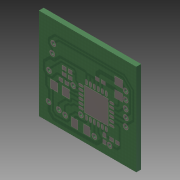
# Autodesk Inventor part: LED_module_PCB
Saved by Autodesk Inventor 2013 (Build 170138000, 138)
## iProperties
Created: 2015-07-03
Part Number: LED_module_PCB
Material: Ogólny
Document SubType Name: Modeling
Designer: terg
Density: 1 g/cm^3
Author: terg
Autodesk Inventor part; units mm, degrees
ref_plane "YZ Plane" through (0, 0, 0) normal (1, 0, 0) x (0, 1, 0)
ref_plane "XZ Plane" through (0, 0, 0) normal (0, 1, 0) x (-1, 0, 0)
ref_plane "XY Plane" through (0, 0, 0) normal (0, 0, 1) x (1, 0, 0)
sketch "Szkic1" plane through (0, 0, 0) normal (0, 1, 0) x (-1, 0, 0)
  line L0 (0, 0) -> (16, 0)
  line L1 (16, 0) -> (16, 15)
  line L2 (16, 15) -> (0, 15)
  line L3 (0, 15) -> (0, 0)
  dimension "d0" = 16
  dimension "d1" = 15
  constraints: 8 end point, 2 parallel, 1 horizontal, 1 perpendicular
  measures "d0" distance of L2.end L1.end
  measures "d1" distance of L1.end L0.end
extrude "Wyciągnięcie proste1" add sketch "Szkic1" along normal blind 0.8
sketch "Szkic2" plane through (0, 0.8, 0) normal (0, 1, 0) x (1, 0, 0)
  line L0 (0, 0) -> (-16, 0) projected
  line L1 (-16, 0) -> (-16, -15) projected
  line L2 (-16, -15) -> (0, -15) projected
  line L3 (0, -15) -> (0, 0) projected
  line L4 (-16.025, 0) -> (0.025, 0) construction
  line L5 (0.025, 0) -> (0.025, -15) construction
  line L6 (0.025, -15) -> (-16.025, -15) construction
  line L7 (-16.025, -15) -> (-16.025, 0) construction
  dimension "d11" = -0.025
  dimension "d12" = 0
  dimension "d13" = 0
  dimension "d14" = -0.025
  constraints: 2 other
  measures "d11" distance between parallel lines of L3 L5
  measures "d12" distance between parallel lines of L0 L4
  measures "d13" distance between parallel lines of L2 L6
  measures "d14" distance between parallel lines of L1 L7
decal "Pokrycie bitmapą1"
sketch "Szkic3" plane through (0, 0, 0) normal (0, -1, 0) x (1, 0, 0)
  line L0 (0, 0) -> (-16, 0) projected
  line L1 (0, 15) -> (0, 0) projected
  line L2 (-16, 15) -> (0, 15) projected
  line L3 (-16, 0) -> (-16, 15) projected
  line L4 (0.0249, 0) -> (-16.0249, 0) construction
  line L5 (-16.0249, 0) -> (-16.0249, 15) construction
  line L6 (-16.0249, 15) -> (0.0249, 15) construction
  line L7 (0.0249, 15) -> (0.0249, 0) construction
  dimension "d28" = 0
  dimension "d29" = 0.0249
  dimension "d30" = 0
  dimension "d31" = 0.0249
  constraints: 2 other
  measures "d28" distance between parallel lines of L0 L4
  measures "d29" distance between parallel lines of L1 L7
  measures "d30" distance between parallel lines of L2 L6
  measures "d31" distance between parallel lines of L3 L5
decal "Pokrycie bitmapą2"
sketch "Szkic4" plane through (0, 0.8, 0) normal (0, 1, 0) x (1, 0, 0)
  point P0 (-14.3793, -2.8439)
  point P1 (-12.7115, -2.5266)
  point P2 (-11.6963, -2.2909)
  point P3 (-9.0949, -3.6143)
  point P4 (-6.8818, -1.6491)
  point P5 (-4.3551, -1.6491)
  point P6 (-1.7394, -5.6091)
  point P7 (-1.6908, -6.9129)
  point P8 (-1.7394, -8.152)
  point P9 (-1.7394, -9.4163)
  point P10 (-1.7394, -10.6891)
  point P11 (-10.3497, -7.1543)
  point P12 (-14.3113, -7.3446)
  point P13 (-13.7882, -10.0071)
  point P14 (-13.6086, -11.5062)
hole "Otwór1" at (-14.3793, 0.8, 2.8439) at (-12.7115, 0.8, 2.5266) at (-11.6963, 0.8, 2.2909) at (-9.0949, 0.8, 3.6143) at (-6.8818, 0.8, 1.6491) at (-4.3551, 0.8, 1.6491) at (-1.7394, 0.8, 5.6091) at (-1.6908, 0.8, 6.9129) at (-1.7394, 0.8, 8.152) at (-1.7394, 0.8, 9.4163) at (-1.7394, 0.8, 10.6891) at (-10.3497, 0.8, 7.1543) at (-14.3113, 0.8, 7.3446) at (-13.7882, 0.8, 10.0071) at (-13.6086, 0.8, 11.5062) direction (0, -1, 0) diameter 0.4 depth 8
equation "\"d11\" = d14"
equation "\"d29\" = d31"
